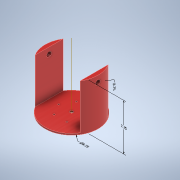
# Autodesk Inventor part: topOfRaBase
Saved by Autodesk Inventor 2021 (Build 250183000, 183)
## iProperties
Created: 2020-05-22
Part Number: topOfRaBase
Material: ABS Plastic
Document SubType Name: Modeling
Designer: robst
Density: 1.06 g/cm^3
Appearance: Orange-Red
Author: robst
Autodesk Inventor part; units mm, degrees
ref_plane "XZ Plane" through (0, 0, 0) normal (0, 1, 0) x (-1, 0, 0)
ref_plane "XY Plane" through (0, 0, 0) normal (0, 0, 1) x (1, 0, 0)
sketch "Sketch1" plane through (0, 0, 0) normal (0, 1, 0) x (-1, 0, 0)
  circle A0 centre (0, 0) radius 104.775
  dimension "baseOutsideDiameter" = 209.55
  constraints: 1 centre point, 1 coincident
  measures "baseOutsideDiameter" diameter of A0
extrude "Extrusion1" add sketch "Sketch1" along normal blind 6.35
sketch "Sketch7" plane through (0, 6.35, 0) normal (0, 1, 0) x (1, 0, 0)
  line L0 (0, 0) -> (0, 104.775) construction
  circle A0 centre (0, 0) radius 104.775 construction
  line L1 (88.9, -55.449) -> (88.9, 55.449)
  arc A1 (88.9, -55.449) -> (88.9, 55.449) centre (0, 0) ccw
  dimension "spaceforTube" = 88.9
  constraints: 5 point on circle, 4 end point, 2 vertical, 1 centre point, 1 coincident, 1 concentric
  measures "spaceforTube" distance from line of L0.start L1
extrude "Extrusion7" add sketch "Sketch7" along normal blind 177.8
mirror "Mirror1" about plane through (0, 0, 0) normal (1, 0, 0) of "Extrusion7"
ref_plane "Work Plane2" through (104.775, 0, 0) normal (1, 0, 0) x (0, 1, 0)
sketch "Sketch8" plane through (104.775, 0, 0) normal (1, 0, 0) x (0, 1, 0)
  circle A0 centre (158.75, 0) radius 9.525
  line L0 (6.35, 55.449) -> (6.35, 104.775) projected
  point P0 (0, 0)
  dimension "d34" = 19.05
  dimension "holeHeight" = 152.4
  constraints: 1 centre point
  measures "d34" diameter of A0
  measures "holeHeight" distance from line of A0.centre L0
extrude "Extrusion8" cut sketch "Sketch8" against normal through all
sketch "Sketch9" plane through (0, 0, 0) normal (0, -1, 0) x (1, 0, 0)
  circle A0 centre (0, 0) radius 6.35
  dimension "d47" = 12.7
  constraints: 1 centre point, 1 coincident
  measures "d47" diameter of A0
extrude "Extrusion9" cut sketch "Sketch9" against normal through all
sketch "Sketch10" plane through (0, 0, 0) normal (0, -1, 0) x (1, 0, 0)
  point P0 (0, 0)
  point P1 (-50.8, 0)
  dimension "d50" = 50.8
  measures "d50" distance of point (-50.8, 0) point (0, 0)
hole "Hole1" at (-50.8, 0, 0) direction (0, 1, 0) diameter 6.7564 end through all clearance for "Socket Head Cap Screw" size "1/4" standard "Ansi Unified Screw Threads"
pattern_circular "Circular Pattern2" count 6 over 360 about axis through (0, -10, 0) along (0, 1, 0) of "Hole1"
equation "\"spaceforTube\" = bracketWidth + 0.5 * tubeDiameter"
equation "\"tubeDiameter\" = 165.1"
equation "\"bracketWidth\" = 6.35"
body "Solid1"
